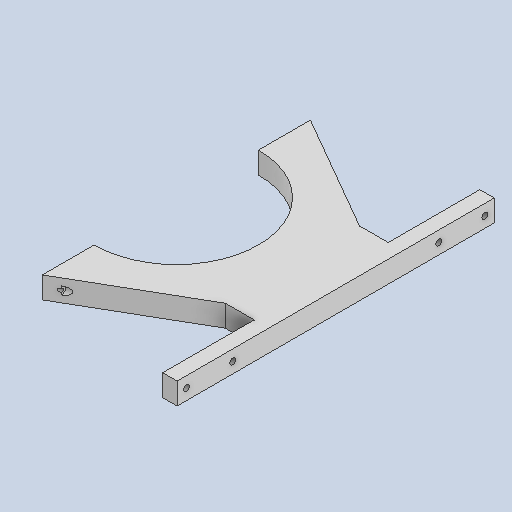
# Autodesk Inventor part: nowtrying
Saved by Autodesk Inventor 2026.3 (Build 303398000, 398)
## iProperties
Created: 2026-06-03
Part Number: nowtrying
Material: 一般
Document SubType Name: Modeling
Designer: shusu
Density: 1 g/cm^3
Appearance: 既定
Author: shusu
Autodesk Inventor part; units mm, degrees
sketch "スケッチ1" plane through (0, 0, 0) normal (0, 1, 0) x (-1, 0, 0)
  arc A0 (0, 57) -> (0, -57) centre (0, 0) ccw
  line L0 (0, 57) -> (0, 93) construction
  line L1 (0, 57) -> (0, 93)
  line L2 (0, 93) -> (-80.5404, 46.5)
  line L3 (-80.5404, 46.5) -> (-100.5404, 46.5)
  line L4 (-100.5404, 46.5) -> (-100.5404, 110)
  line L5 (-100.5404, 110) -> (-110.5404, 110)
  line L6 (-110.5404, 110) -> (-110.5404, 0)
  line L7 (0, -57) -> (0, -93) construction
  line L8 (0, -93) -> (-80.5404, -46.5)
  line L9 (-80.5404, -46.5) -> (-100.5404, -46.5)
  line L10 (-100.5404, -46.5) -> (-100.5404, -110)
  line L11 (-100.5404, -110) -> (-110.5404, -110)
  line L12 (-110.5404, -110) -> (-110.5404, 0)
  line L13 (0, -93) -> (0, -57)
  dimension "d0" = 57
  dimension "d7" = 10
  constraints: 28 end point, 2 collinear, 2 perpendicular, 2 point on circle, 1 centre point, 1 coincident, 1 horizontal, 1 vertical
  measures "d0" radius of A0
  measures "d7" distance of L4.end L5.end
sketch "スケッチ2" plane through (0, 0, 0) normal (0, 1, 0) x (-1, 0, 0)
  point P0 (0, 0)
extrude "押し出し1" add sketch "スケッチ1" along normal blind 15
sketch "スケッチ3" plane through (100.5404, 0, 46.5) normal (-1, 0, 0) x (0, 0, 1)
  point P0 (-46.5, 0)
sketch "スケッチ4" plane through (0, 0, 57) normal (-1, 0, 0) x (0, 0, 1)
  line L0 (0, 0) -> (0, 15) projected
  line L1 (0, 0) -> (31, 0)
  line L2 (36, 0) -> (36, 15) projected
  line L3 (31, 0) -> (31, 7.5)
  point P0 (-57, 0)
  dimension "d10" = 31
  dimension "d11" = 7.5
  constraints: 4 end point, 2 perpendicular
  measures "d10" distance of L0.start L1.end
  measures "d11" distance of L1.end L3.end
hole "穴1" at (0, 7.5, 88) direction (1, 0, 0) diameter 2.459 depth 31.54 tip angle 118 thread size "M3x0.5" class "6H" standard "ISO Metric profile"
sketch "スケッチ5" plane through (0, 0, -93) normal (-1, 0, 0) x (0, 0, 1)
  line L0 (36, 0) -> (36, 15) projected
  line L1 (36, 0) -> (5, 0)
  line L2 (-17, 0) -> (46.5, 0) projected
  line L3 (5, 0) -> (5, 7.5)
  line L4 (-17, 15) -> (46.5, 15) projected
  point P0 (93, 0)
  dimension "d19" = 31
  dimension "d20" = 7.5
  constraints: 4 end point, 1 perpendicular, 1 point on line
  measures "d19" distance of L0.start L1.end
  measures "d20" distance of L1.end L3.end
hole "穴2" at (0, 7.5, -88) direction (1, 0, 0) diameter 2.459 depth 35.79 tip angle 118 thread size "M3x0.5" class "6H" standard "ISO Metric profile"
sketch "スケッチ7" plane through (0, 0, -93) normal (0.5, 0, -0.866) x (-0.866, 0, -0.5)
  ellipse E0 centre (-10, 7.5) end of major axis (-12.459, 7.5) minor radius 1.2295 projected
  point P0 (-46.5, 0)
  point P1 (-10, 7.5)
  constraints: 1 coincident, 1 other
ref_plane "作業平面1" through (8.6603, 7.5, -88) normal (0, 0, 1) x (1, 0, 0)
sketch "スケッチ8" plane through (8.6603, 7.5, -88) normal (0, 0, 1) x (1, 0, 0)
  ellipse E0 centre (0, 0) end of major axis (-2.1296, 0) minor radius 1.2295 projected
  line L0 (0, 0) -> (4.8, 0)
  point P0 (-8.6603, -7.5)
  dimension "d28" = 4.8
  constraints: 2 end point, 1 horizontal, 1 other
  measures "d28" distance of L0.start L0.end
ref_plane "作業平面2" through (13.4603, 7.5, -88) normal (-1, 0, 0) x (0, 0, 1)
sketch "スケッチ9" plane through (13.4603, 7.5, -88) normal (-1, 0, 0) x (0, 0, 1)
  point P0 (88, -7.5)
  point P1 (0, 0)
hole "穴3" at (13.4603, 7.5, -88) direction (-1, 0, 0) diameter 2.459 end through all counterbore diameter 5.5 counterbore depth 5 thread size "M3x0.5" class "6H" standard "ISO Metric profile"
sketch "スケッチ10" plane through (100.5404, 0, 46.5) normal (-1, 0, 0) x (0, 0, 1)
  line L0 (63.5, 0) -> (63.5, 15) projected
  line L1 (63.5, 7.5) -> (57, 7.5)
  line L2 (46.5, 0) -> (46.5, 15) projected
  line L3 (57, 7.5) -> (25, 7.5)
  point P0 (-46.5, 0)
  dimension "d36" = 6.5
  dimension "d37" = 32
  constraints: 4 end point, 2 coincident, 2 perpendicular, 1 midpoint
  measures "d36" distance of L1.start L1.end
  measures "d37" distance of L3.start L3.end
hole "穴4" at (100.5404, 7.5, 103.5) at (100.5404, 7.5, 71.5) direction (1, 0, 0) diameter 4.134 end through all counterbore diameter 9 counterbore depth 1 thread size "M5x0.8" class "6H" standard "ISO Metric profile"
ref_plane "作業平面3" through (0, 0, 0) normal (0, 0, 1) x (1, 0, 0)
mirror "ミラー1" about plane through (0, 0, 0) normal (0, 0, 1) of "穴4", "穴3"
